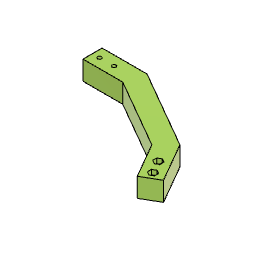
assembly (Autodesk Fusion 360 archive; units mm, degrees)
design "circular_frame"
Autodesk Fusion 360 part; units mm, degrees
(part 1 of 2)
sketch "Sketch1" plane through (0, 0, 0) normal (0, 0, 1) x (1, 0, 0)
  line L0 (151.5544, -62.5) -> (128.1089, -21.8911)
  line L1 (128.1089, -21.8911) -> (46.8911, 25)
  line L2 (46.8911, 25) -> (0, 25)
  line L3 (0, 0) -> (0, 25)
  arc A0 (129.9038, -75) -> (0, 0) centre (0, -150) ccw
  line L4 (151.5544, -62.5) -> (129.9038, -75)
  line L5 (113.4679, -36.5321) -> (41.5321, 5)
  line L6 (41.5321, 5) -> (0, 5)
  line L7 (134.2339, -72.5) -> (113.4679, -36.5321)
  line L8 (77.5, -15.7661) -> (87.5, 1.5544)
  point P0 (0, -150)
  point P1 (0, -150)
  dimension "d1" = 300
  dimension "d4" = 150
  dimension "d5" = 150
  dimension "d14" = 25
  dimension "d15" = 25
  dimension "d16" = 60
  dimension "d17" = 175
  dimension "d30" = 20
  dimension "d31" = 20
  dimension "d32" = 20
  constraint coincident L3.start A0
  constraint vertical L3.start A0.centre
  constraint coincident P0 A0.centre
  constraint horizontal L2
  constraint coincident L3.start A0.end
  constraint coincident L3 A0.end
  constraint collinear L3.start P1 L2.end
  constraint collinear P0 L0.start A0.start
  constraint coincident L3 L6.end
  constraint perpendicular L3 L6
  constraint parallel L1 L5
  constraint midpoint L5 L8.start
  constraint midpoint L1 L8.end
  measures "d1" diameter of A0
  measures "d4" angle of L1 L2
  measures "d5" angle of L0 L1
  measures "d14" distance of L3.start L2.end
  measures "d15" distance of L0.start A0.start
  measures "d16" angle of L3 L4
  measures "d17" distance of P0 L1
  measures "d30" distance of L0 L7
  measures "d31" distance of L2.end L6.end
  measures "d32" distance of L1 L5
extrude "Extrude1" add sketch "Sketch1" along normal blind 20 contours L1 L2 L3 L5 L6 L8
mirror "Mirror2" about plane through (77.5, -15.7661, 0) normal (0.866025, -0.5, 0) of bodies 1 merged
sketch "Sketch4" plane through (0, 0, 20) normal (0, 0, 1) x (-1, 0, 0)
  line L0 (-128.1089, 21.8911) -> (-46.8911, -25)
  line L1 (-46.8911, -25) -> (0, -25)
  line L2 (-41.5321, -5) -> (-41.5321, -25) construction
  line L3 (-41.5321, -15) -> (0, -15) construction
  circle A0 centre (-7.5, -15) radius 2
  circle A1 centre (-22.5, -15) radius 2
  line L4 (-3.8, -17.1362) -> (-3.8, -12.8638)
  line L5 (-3.8, -12.8638) -> (-7.5, -10.7276)
  line L6 (-7.5, -10.7276) -> (-11.2, -12.8638)
  line L7 (-11.2, -12.8638) -> (-11.2, -17.1362)
  line L8 (-11.2, -17.1362) -> (-7.5, -19.2724)
  line L9 (-7.5, -19.2724) -> (-3.8, -17.1362)
  line L10 (-18.8, -17.1362) -> (-18.8, -12.8638)
  line L11 (-18.8, -12.8638) -> (-22.5, -10.7276)
  line L12 (-22.5, -10.7276) -> (-26.2, -12.8638)
  line L13 (-26.2, -12.8638) -> (-26.2, -17.1362)
  line L14 (-26.2, -17.1362) -> (-22.5, -19.2724)
  line L15 (-22.5, -19.2724) -> (-18.8, -17.1362)
  line L16 (0, -5) -> (-41.5321, -5)
  line L17 (-41.5321, -5) -> (-113.4679, 36.5321)
  line L18 (0, -25) -> (0, -5)
  line L19 (-113.4679, 36.5321) -> (-134.2339, 72.5)
  line L20 (-134.2339, 72.5) -> (-151.5544, 62.5)
  line L21 (-151.5544, 62.5) -> (-128.1089, 21.8911)
  line L22 (-77.5, 15.7661) -> (-87.5, -1.5544) construction
  line L23 (-142.8442, 58.8686) -> (-142.8442, 63.141)
  line L24 (-139.1442, 56.7324) -> (-142.8442, 58.8686)
  line L25 (-135.4442, 58.8686) -> (-139.1442, 56.7324)
  line L26 (-135.4442, 63.141) -> (-135.4442, 58.8686)
  line L27 (-139.1442, 65.2772) -> (-135.4442, 63.141)
  line L28 (-142.8442, 63.141) -> (-139.1442, 65.2772)
  line L29 (-131.6442, 52.2868) -> (-127.9442, 50.1506)
  line L30 (-135.3442, 50.1506) -> (-131.6442, 52.2868)
  line L31 (-135.3442, 45.8782) -> (-135.3442, 50.1506)
  line L32 (-131.6442, 43.742) -> (-135.3442, 45.8782)
  line L33 (-127.9442, 45.8782) -> (-131.6442, 43.742)
  line L34 (-127.9442, 50.1506) -> (-127.9442, 45.8782)
  circle A2 centre (-139.1442, 61.0048) radius 2
  circle A3 centre (-131.6442, 48.0144) radius 2
  point P0 (-7.5, -15)
  point P1 (-22.5, -15)
  dimension "d18" = 4
  dimension "d19" = 7.5
  dimension "d20" = 15
  dimension "d21" = 7.4
  constraint coincident L1 L2.end
  constraint perpendicular L1 L2
  constraint midpoint L2 L3.start
  constraint coincident L3 P0
  constraint coincident L3 P1
  constraint equal A0 A1
  constraint coincident P0 A0.centre
  constraint coincident P1 A1.centre
  constraint vertical L4
  constraint vertical L10
  constraint horizontal L8.end L14.end
  constraint horizontal L3
  constraint coincident L2.start L16
  constraint coincident L3.end L18
  constraint coincident L2.start L16.end
  constraint midpoint L17 L22.start
  constraint midpoint L0 L22.end
  constraint symmetric L4.start L22 L23.end
  constraint symmetric L4.end L22 L27.start
  constraint symmetric L5.end L22 L26.start
  constraint symmetric L6.end L22 L25.start
  constraint symmetric L7.end L22 L24.start
  constraint symmetric L8.end L22 L23.start
  constraint symmetric L10.start L22 L30.start
  constraint symmetric L10.end L22 L29.start
  constraint symmetric L11.end L22 L29.end
  constraint symmetric L12.end L22 L33.start
  constraint symmetric L13.end L22 L32.start
  constraint symmetric L14.end L22 L31.start
  constraint symmetric A0 L22 A2
  constraint symmetric A1 L22 A3
  measures "d18" diameter of A0
  measures "d19" distance of L3.end P0
  measures "d20" distance of P0 P1
  measures "d21" distance of L4 L7
extrude "Extrude4" cut sketch "Sketch4" against normal through all contours A0 | A1 | A2 | A3
extrude "Extrude5" cut sketch "Sketch4" along normal blind 5 from surface at -20 contours L4 L5 L6 L7 L8 L9 | L10 L11 L12 L13 L14 L15
extrude "Extrude6" cut sketch "Sketch4" against normal blind 5 contours L23 L24 L25 L26 L27 L28 | L29 L30 L31 L32 L33 L34
equation "d21 = 7 mm + 2 * gap"
equation "gap = 0.2 mm"

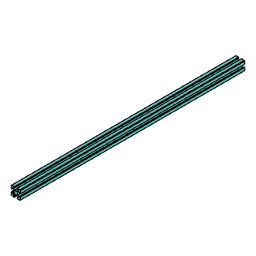
design "profile"
Autodesk Fusion 360 part; units mm, degrees
sketch "Sketch1" plane through (0, 0, 0) normal (0, 1, 0) x (1, 0, 0)
  line L0 (3.5, 0) -> (3.5, -2.7929)
  line L1 (3.5, -2.7929) -> (5.7071, -5)
  line L2 (5.7071, -5) -> (8, -5)
  line L3 (10, -3) -> (10, -10)
  line L4 (0, 0) -> (10, -10)
  line L5 (3.5, 0) -> (0, 0)
  line L6 (8, -5) -> (8, -3)
  line L7 (8, -3) -> (10, -3)
  dimension "d4" = 45
  dimension "d5" = 0.5
  dimension "d7" = 7
  dimension "d8" = 2
  dimension "d9" = 2
  dimension "d10" = 3.5
  dimension "d11" = 10
  constraint vertical L0
  constraint perpendicular L0 L2
  constraint perpendicular L2 L3
  constraint coincident L4.start L5.end
  constraint perpendicular L0 L5
  constraint parallel L1 L4
  constraint perpendicular L2 L6
  constraint horizontal L7
  measures "d4" angle of L4 L5
  measures "d5" distance of L1 L4
  measures "d7" distance of L3.start L3.end
  measures "d8" distance of L2.end L6.end
  measures "d9" distance of L3.start L6.end
  measures "d10" distance of L0.start L4.start
  measures "d11" distance of L4.start L3
extrude "Extrude1" add sketch "Sketch1" along normal blind 490
mirror "Mirror1" about plane through (0, 0, 0) normal (-0.707107, 0, 0.707107) of bodies 1 merged
mirror "Mirror2" about plane through (0, 0, 3.5) normal (-1, 0, 0) of bodies 1 merged
mirror "Mirror3" about plane through (3.5, 0, 0) normal (0, 0, -1) of bodies 1 merged
fillet "Fillet1" radius 1 4 edges at (-10, 245, 10) (10, 245, 10) (-10, 245, -10) (10, 245, -10)
sketch "Sketch2" plane through (0, 0, 0) normal (0, -1, 0) x (1, 0, 0)
  arc A0 (9, -10) -> (10, -9) centre (9, -9) ccw
  line L0 (10, -9) -> (10, -3)
  line L1 (10, -3) -> (8, -3)
  line L2 (8, -3) -> (8, -5)
  line L3 (8, -5) -> (5.7071, -5)
  line L4 (5.7071, -5) -> (3.5, -2.7929)
  line L5 (3.5, -2.7929) -> (3.5, 2.7929)
  line L6 (3.5, 2.7929) -> (5.7071, 5)
  line L7 (5.7071, 5) -> (8, 5)
  line L8 (8, 5) -> (8, 3)
  line L9 (8, 3) -> (10, 3)
  line L10 (10, 3) -> (10, 9)
  arc A1 (10, 9) -> (9, 10) centre (9, 9) ccw
  line L11 (9, 10) -> (3, 10)
  line L12 (3, 10) -> (3, 8)
  line L13 (3, 8) -> (5, 8)
  line L14 (5, 8) -> (5, 5.7071)
  line L15 (5, 5.7071) -> (2.7929, 3.5)
  line L16 (2.7929, 3.5) -> (-2.7929, 3.5)
  line L17 (-2.7929, 3.5) -> (-5, 5.7071)
  line L18 (-5, 5.7071) -> (-5, 8)
  line L19 (-5, 8) -> (-3, 8)
  line L20 (-3, 8) -> (-3, 10)
  line L21 (-3, 10) -> (-9, 10)
  arc A2 (-9, 10) -> (-10, 9) centre (-9, 9) ccw
  line L22 (-10, 9) -> (-10, 3)
  line L23 (-10, 3) -> (-8, 3)
  line L24 (-8, 3) -> (-8, 5)
  line L25 (-8, 5) -> (-5.7071, 5)
  line L26 (-5.7071, 5) -> (-3.5, 2.7929)
  line L27 (-3.5, 2.7929) -> (-3.5, -2.7929)
  line L28 (-3.5, -2.7929) -> (-5.7071, -5)
  line L29 (-5.7071, -5) -> (-8, -5)
  line L30 (-8, -5) -> (-8, -3)
  line L31 (-8, -3) -> (-10, -3)
  line L32 (-10, -3) -> (-10, -9)
  arc A3 (-10, -9) -> (-9, -10) centre (-9, -9) ccw
  line L33 (-9, -10) -> (-3, -10)
  line L34 (-3, -10) -> (-3, -8)
  line L35 (-3, -8) -> (-5, -8)
  line L36 (-5, -8) -> (-5, -5.7071)
  line L37 (-5, -5.7071) -> (-2.7929, -3.5)
  line L38 (-2.7929, -3.5) -> (2.7929, -3.5)
  line L39 (2.7929, -3.5) -> (5, -5.7071)
  line L40 (5, -5.7071) -> (5, -8)
  line L41 (5, -8) -> (3, -8)
  line L42 (3, -8) -> (3, -10)
  line L43 (3, -10) -> (9, -10)
  line L44 (2.9, 7.9) -> (4.9, 7.9)
  line L45 (4.9, 7.9) -> (4.9, 5.7485)
  line L46 (4.9, 5.7485) -> (2.7515, 3.6)
  line L47 (2.7515, 3.6) -> (-2.7515, 3.6)
  line L48 (-2.7515, 3.6) -> (-4.9, 5.7485)
  line L49 (-4.9, 5.7485) -> (-4.9, 7.9)
  line L50 (-4.9, 7.9) -> (-2.9, 7.9)
  line L51 (-2.9, 7.9) -> (-2.9, 10.1)
  line L52 (-2.9, 10.1) -> (-9, 10.1)
  arc A4 (-9, 10.1) -> (-10.1, 9) centre (-9, 9) ccw
  line L53 (-10.1, 9) -> (-10.1, 2.9)
  line L54 (-10.1, 2.9) -> (-7.9, 2.9)
  line L55 (-7.9, 2.9) -> (-7.9, 4.9)
  line L56 (-7.9, 4.9) -> (-5.7485, 4.9)
  line L57 (-5.7485, 4.9) -> (-3.6, 2.7515)
  line L58 (-3.6, 2.7515) -> (-3.6, -2.7515)
  line L59 (-3.6, -2.7515) -> (-5.7485, -4.9)
  line L60 (-5.7485, -4.9) -> (-7.9, -4.9)
  line L61 (-7.9, -4.9) -> (-7.9, -2.9)
  line L62 (-7.9, -2.9) -> (-10.1, -2.9)
  line L63 (-10.1, -2.9) -> (-10.1, -9)
  arc A5 (-10.1, -9) -> (-9, -10.1) centre (-9, -9) ccw
  line L64 (-9, -10.1) -> (-2.9, -10.1)
  line L65 (-2.9, -10.1) -> (-2.9, -7.9)
  line L66 (-2.9, -7.9) -> (-4.9, -7.9)
  line L67 (-4.9, -7.9) -> (-4.9, -5.7485)
  line L68 (-4.9, -5.7485) -> (-2.7515, -3.6)
  line L69 (-2.7515, -3.6) -> (2.7515, -3.6)
  line L70 (2.7515, -3.6) -> (4.9, -5.7485)
  line L71 (4.9, -5.7485) -> (4.9, -7.9)
  line L72 (4.9, -7.9) -> (2.9, -7.9)
  line L73 (2.9, -7.9) -> (2.9, -10.1)
  line L74 (2.9, -10.1) -> (9, -10.1)
  arc A6 (9, -10.1) -> (10.1, -9) centre (9, -9) ccw
  line L75 (10.1, -9) -> (10.1, -2.9)
  line L76 (10.1, -2.9) -> (7.9, -2.9)
  line L77 (7.9, -2.9) -> (7.9, -4.9)
  line L78 (7.9, -4.9) -> (5.7485, -4.9)
  line L79 (5.7485, -4.9) -> (3.6, -2.7515)
  line L80 (3.6, -2.7515) -> (3.6, 2.7515)
  line L81 (3.6, 2.7515) -> (5.7485, 4.9)
  line L82 (5.7485, 4.9) -> (7.9, 4.9)
  line L83 (7.9, 4.9) -> (7.9, 2.9)
  line L84 (7.9, 2.9) -> (10.1, 2.9)
  line L85 (10.1, 2.9) -> (10.1, 9)
  arc A7 (10.1, 9) -> (9, 10.1) centre (9, 9) ccw
  line L86 (9, 10.1) -> (2.9, 10.1)
  line L87 (2.9, 10.1) -> (2.9, 7.9)
  dimension "d22" = 0.1
sketch "Sketch3" plane through (0, 0, 0) normal (0, 1, 0) x (1, 0, 0)
  line L0 (10.1, 9) -> (10.1, 2.9)
  arc A0 (10.1, 9) -> (9, 10.1) centre (9, 9) ccw
  line L1 (2.9, 10.1) -> (9, 10.1)
  line L2 (2.9, 7.9) -> (2.9, 10.1)
  line L3 (4.9, 7.9) -> (2.9, 7.9)
  line L4 (4.9, 5.7485) -> (4.9, 7.9)
  line L5 (2.7515, 3.6) -> (4.9, 5.7485)
  line L6 (5.7485, 4.9) -> (3.6, 2.7515)
  line L7 (7.9, 4.9) -> (5.7485, 4.9)
  line L8 (7.9, 2.9) -> (7.9, 4.9)
  line L9 (10.1, 2.9) -> (7.9, 2.9)
  line L10 (3.6, 2.7515) -> (3.6, -2.7515)
  line L11 (3.6, -2.7515) -> (5.7485, -4.9)
  line L12 (5.7485, -4.9) -> (7.9, -4.9)
  line L13 (7.9, -4.9) -> (7.9, -2.9)
  line L14 (7.9, -2.9) -> (10.1, -2.9)
  line L15 (10.1, -2.9) -> (10.1, -9)
  arc A1 (9, -10.1) -> (10.1, -9) centre (9, -9) ccw
  line L16 (9, -10.1) -> (2.9, -10.1)
  line L17 (2.9, -10.1) -> (2.9, -7.9)
  line L18 (2.9, -7.9) -> (4.9, -7.9)
  line L19 (4.9, -7.9) -> (4.9, -5.7485)
  line L20 (4.9, -5.7485) -> (2.7515, -3.6)
  line L21 (2.7515, -3.6) -> (-2.7515, -3.6)
  line L22 (-2.7515, -3.6) -> (-4.9, -5.7485)
  line L23 (-4.9, -5.7485) -> (-4.9, -7.9)
  line L24 (-4.9, -7.9) -> (-2.9, -7.9)
  line L25 (-2.9, -7.9) -> (-2.9, -10.1)
  line L26 (-2.9, -10.1) -> (-9, -10.1)
  arc A2 (-10.1, -9) -> (-9, -10.1) centre (-9, -9) ccw
  line L27 (-10.1, -9) -> (-10.1, -2.9)
  line L28 (-10.1, -2.9) -> (-7.9, -2.9)
  line L29 (-7.9, -2.9) -> (-7.9, -4.9)
  line L30 (-7.9, -4.9) -> (-5.7485, -4.9)
  line L31 (-5.7485, -4.9) -> (-3.6, -2.7515)
  line L32 (-3.6, -2.7515) -> (-3.6, 2.7515)
  line L33 (-3.6, 2.7515) -> (-5.7485, 4.9)
  line L34 (-7.9, 2.9) -> (-10.1, 2.9)
  line L35 (-7.9, 4.9) -> (-7.9, 2.9)
  line L36 (-5.7485, 4.9) -> (-7.9, 4.9)
  line L37 (-10.1, 2.9) -> (-10.1, 9)
  line L38 (-4.9, 5.7485) -> (-2.7515, 3.6)
  line L39 (-2.7515, 3.6) -> (2.7515, 3.6)
  line L40 (-4.9, 7.9) -> (-4.9, 5.7485)
  line L41 (-2.9, 7.9) -> (-4.9, 7.9)
  line L42 (-2.9, 10.1) -> (-2.9, 7.9)
  line L43 (-9, 10.1) -> (-2.9, 10.1)
  arc A3 (-9, 10.1) -> (-10.1, 9) centre (-9, 9) ccw

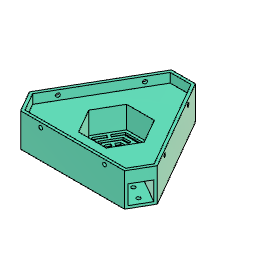
design "lower_connector"
Autodesk Fusion 360 part; units mm, degrees
sketch "Sketch1" plane through (0, 0, 0) normal (0, 0, 1) x (1, 0, 0)
  line L0 (-26, 0) -> (-82.282, -97.4833)
  line L1 (-69.282, -120) -> (43.282, -120)
  line L2 (56.282, -97.4833) -> (0, 0)
  line L3 (49.782, -108.7417) -> (-54.141, -48.7417) construction
  line L4 (0, 0) -> (-26, 0)
  line L5 (-82.282, -97.4833) -> (-69.282, -120)
  line L6 (43.282, -120) -> (56.282, -97.4833)
  line L7 (-13, 0) -> (-13, -120) construction
  line L8 (-75.782, -108.7417) -> (28.141, -48.7417) construction
  line L9 (-24.2679, -3) -> (-78.8179, -97.4833)
  line L10 (-78.8179, -97.4833) -> (-67.55, -117)
  line L11 (-67.55, -117) -> (41.55, -117)
  line L12 (41.55, -117) -> (52.8179, -97.4833)
  line L13 (52.8179, -97.4833) -> (-1.7321, -3)
  line L14 (-1.7321, -3) -> (-24.2679, -3)
  line L15 (2, -98.4752) -> (-28, -98.4752)
  line L16 (-28, -98.4752) -> (-43, -72.4944)
  line L17 (-43, -72.4944) -> (-28, -46.5137)
  line L18 (-28, -46.5137) -> (2, -46.5137)
  line L19 (2, -46.5137) -> (17, -72.4944)
  line L20 (17, -72.4944) -> (2, -98.4752)
  point P0 (-13, -72.4944)
  dimension "d18" = 120
  dimension "d25" = -3
  dimension "d36" = 26
  dimension "d42" = 30
  constraint coincident L2.end L4.start
  constraint horizontal L1
  constraint midpoint L0 L3.end
  constraint coincident L3 P0
  constraint symmetric L1.end L2.start L3
  constraint coincident L3.start L6
  constraint horizontal L4
  constraint midpoint L4 L7.start
  constraint midpoint L1 L7.end
  constraint midpoint L5 L8.start
  constraint midpoint L2 L8.end
  constraint coincident P0 L8
  constraint coincident P0 L7
  constraint perpendicular L4 L7
  constraint perpendicular L5 L8
  constraint symmetric L0 L1 L8
  constraint symmetric L0 L2 L7
  constraint equal L1 L2
  constraint horizontal L15
  constraint perpendicular L8 L16
  constraint parallel L15 L18
  constraint perpendicular L3 L20
  constraint perpendicular L8 L19
  constraint perpendicular L3 L17
  constraint symmetric L7 L16 L20
  constraint symmetric L7 L17 L19
  constraint symmetric L3 L16 L18
  constraint symmetric L3 L15 L19
  constraint equal L15 L16
  measures "d18" distance of L2.end L1
  measures "d36" distance of L1.end L2.start
  measures "d42" distance of L15.start L15.end
extrude "Extrude7" add sketch "Sketch1" along normal blind 2 contours L15 L16 L17 L18 L19 L20
extrude "Extrude4" add sketch "Sketch1" along normal blind 26 contours L0 L1 L2 L4 L5 L6 | L9 L10 L11 L12 L13 L14
sketch "Sketch2" plane through (84.423, -48.7417, 0) normal (0.866025, -0.5, 0) x (0.5, 0.866025, 0)
  line L0 (-82.282, 0) -> (-56.282, 0)
  line L1 (-56.282, 0) -> (-56.282, 26)
  line L2 (-56.282, 26) -> (-82.282, 26)
  line L3 (-82.282, 26) -> (-82.282, 0)
  line L4 (-82.282, 0) -> (-56.282, 26) construction
  line L5 (-56.282, 0) -> (-82.282, 26) construction
  line L6 (-79.482, 2.8) -> (-59.082, 2.8)
  line L7 (-59.082, 2.8) -> (-59.082, 23.2)
  line L8 (-59.082, 23.2) -> (-79.482, 23.2)
  line L9 (-79.482, 23.2) -> (-79.482, 2.8)
  dimension "d79" = 20.4
  constraint coincident L0.start L3.end
  constraint coincident L1.end L2.start
  constraint coincident L0.end L1.start
  constraint coincident L2.end L3.start
  constraint horizontal L6
  constraint vertical L7
  constraint horizontal L8
  constraint vertical L9
  constraint coincident L4 L7.end
  constraint coincident L4 L6.start
  constraint coincident L5 L8.end
  measures "d79" distance of L7.end L8.end
extrude "Extrude5" cut sketch "Sketch2" against normal blind 30 contours L6 L7 L8 L9
sketch "Sketch8" plane through (0, 0, 0) normal (0, 1, 0) x (-1, 0, 0)
  line L0 (0, 0) -> (26, 0)
  line L1 (26, 0) -> (26, 26)
  line L2 (26, 26) -> (0, 26)
  line L3 (0, 26) -> (0, 0)
  line L4 (0, 0) -> (26, 26) construction
  line L5 (0, 26) -> (26, 0) construction
  line L6 (2.8, 2.8) -> (23.2, 2.8)
  line L7 (23.2, 2.8) -> (23.2, 23.2)
  line L8 (23.2, 23.2) -> (2.8, 23.2)
  line L9 (2.8, 23.2) -> (2.8, 2.8)
  dimension "d62" = 20.4
  constraint coincident L0.start L3.end
  constraint coincident L1.end L2.start
  constraint coincident L2.end L3.start
  constraint coincident L0.end L1.start
  constraint horizontal L6
  constraint vertical L7
  constraint horizontal L8
  constraint vertical L9
  constraint coincident L4 L7.end
  constraint coincident L4 L6.start
  constraint coincident L5 L8.end
  measures "d62" distance of L7.end L8.end
extrude "Extrude9" cut sketch "Sketch8" against normal blind 30 contours L6 L7 L8 L9
sketch "Sketch9" plane through (-103.923, -60, 0) normal (-0.866025, -0.5, 0) x (0.5, -0.866025, 0)
  line L0 (43.282, 0) -> (69.282, 0)
  line L1 (69.282, 0) -> (69.282, 26)
  line L2 (69.282, 26) -> (43.282, 26)
  line L3 (43.282, 26) -> (43.282, 0)
  line L4 (43.282, 0) -> (69.282, 26) construction
  line L5 (43.282, 26) -> (69.282, 0) construction
  line L6 (46.082, 2.8) -> (66.482, 2.8)
  line L7 (66.482, 2.8) -> (66.482, 23.2)
  line L8 (66.482, 23.2) -> (46.082, 23.2)
  line L9 (46.082, 23.2) -> (46.082, 2.8)
  dimension "d65" = 20.4
  constraint coincident L0.start L3.end
  constraint coincident L1.end L2.start
  constraint coincident L2.end L3.start
  constraint coincident L0.end L1.start
  constraint horizontal L6
  constraint vertical L7
  constraint horizontal L8
  constraint vertical L9
  constraint coincident L4 L7.end
  constraint coincident L4 L6.start
  constraint coincident L5 L8.end
  measures "d65" distance of L7.end L8.end
extrude "Extrude10" cut sketch "Sketch9" against normal blind 30 contours L6 L7 L8 L9
sketch "Sketch7" plane through (0, 0, 2) normal (0, 0, 1) x (-1, 0, 0)
  line L0 (14.5, 80.4752, 24) -> (14.5, 83.4752, 24)
  line L1 (17.6077, 80.4752, 24) -> (14.5, 80.4752, 24)
  line L2 (24.3577, 80.7839, 24) -> (26.9558, 82.2839, 24)
  line L3 (18.7513, 72.4944, 24) -> (18.0635, 73.6858, 24)
  line L4 (25.6795, 72.4944, 24) -> (19.3397, 83.4752, 24)
  line L5 (22.2154, 72.4944, 24) -> (20.6615, 75.1858, 24)
  line L6 (19.1615, 77.7839, 24) -> (17.6077, 80.4752, 24)
  line L7 (24.3577, 80.7839, 24) -> (21.0718, 86.4752, 24)
  line L8 (20.6615, 75.1858, 24) -> (19.1615, 77.7839, 24)
  line L9 (19.3397, 83.4752, 24) -> (14.5, 83.4752, 24)
  line L10 (18.0635, 73.6858, 24) -> (20.6615, 75.1858, 24)
  line L11 (25.8577, 78.1858, 24) -> (28.4558, 79.6858, 24)
  line L12 (16.5635, 76.2839, 24) -> (15.8756, 77.4752, 24)
  line L13 (18.0635, 73.6858, 24) -> (16.5635, 76.2839, 24)
  line L14 (15.8756, 77.4752, 24) -> (10.1244, 77.4752, 24)
  line L15 (16.5635, 76.2839, 24) -> (19.1615, 77.7839, 24)
  line L16 (26.2679, 95.4752, 24) -> (14.5, 95.4752, 24)
  line L17 (24.5359, 92.4752, 24) -> (14.5, 92.4752, 24)
  line L18 (29.1436, 72.4944, 24) -> (25.8577, 78.1858, 24)
  line L19 (6.6603, 61.5137, 24) -> (19.3397, 61.5137, 24)
  line L20 (26.9558, 82.2839, 24) -> (22.8038, 89.4752, 24)
  line L21 (14.5, 58.5137, 24) -> (21.0718, 58.5137, 24)
  line L22 (14.5, 55.5137, 24) -> (22.8038, 55.5137, 24)
  line L23 (11.5, 64.5137, 24) -> (14.5, 64.5137, 24)
  line L24 (14.5, 92.4752, 24) -> (14.5, 95.4752, 24)
  line L25 (19.3397, 61.5137, 24) -> (21.7596, 65.705, 24)
  line L26 (17.6077, 64.5137, 24) -> (19.1615, 67.205, 24)
  line L27 (32.6077, 72.4944, 24) -> (28.4558, 79.6858, 24)
  line L28 (34.75, 58.205, 24) -> (-10.25, 84.1858, 24) construction
  line L29 (4.2404, 65.705, 24) -> (2.7404, 68.3031, 24)
  line L30 (3.1962, 55.5137, 24) -> (11.5, 55.5137, 24)
  line L31 (10.1244, 67.5137, 24) -> (11.5, 67.5137, 24)
  line L32 (5.3385, 69.8031, 24) -> (2.7404, 68.3031, 24)
  line L33 (3.7846, 72.4944, 24) -> (5.3385, 69.8031, 24)
  line L34 (7.2487, 72.4944, 24) -> (10.1244, 67.5137, 24)
  line L35 (-0.2679, 49.5137, 24) -> (26.2679, 49.5137, 24)
  line L36 (0.3205, 72.4944, 24) -> (2.7404, 68.3031, 24)
  line L37 (6.8385, 67.205, 24) -> (5.3385, 69.8031, 24)
  line L38 (-13.5359, 72.4944, 24) -> (-7.6519, 62.3031, 24)
  line L39 (-2, 46.5137, 24) -> (28, 46.5137, 24)
  line L40 (-2, 98.4752, 24) -> (-17, 72.4944, 24)
  line L41 (11.5, 98.4752, 24) -> (11.5, 46.5137, 24) construction
  line L42 (-6.6077, 72.4944, 24) -> (3.1962, 55.5137, 24)
  line L43 (-17, 72.4944, 24) -> (-2, 46.5137, 24)
  line L44 (11.5, 67.5137, 24) -> (11.5, 64.5137, 24)
  line L45 (8.3923, 64.5137, 24) -> (11.5, 64.5137, 24)
  line L46 (34.75, 86.7839, 24) -> (-10.25, 60.8031, 24) construction
  line L47 (11.5, 58.5137, 24) -> (11.5, 55.5137, 24)
  line L48 (4.2404, 65.705, 24) -> (6.6603, 61.5137, 24)
  line L49 (6.8385, 67.205, 24) -> (4.2404, 65.705, 24)
  line L50 (6.8385, 67.205, 24) -> (8.3923, 64.5137, 24)
  line L51 (-3.5538, 61.205, 24) -> (1.4641, 52.5137, 24)
  line L52 (-9.5, 59.5041, 24) -> (35.5, 85.4848, 24) construction
  line L53 (4.9282, 58.5137, 24) -> (11.5, 58.5137, 24)
  line L54 (-10.0718, 72.4944, 24) -> (-5.0538, 63.8031, 24)
  line L55 (36.25, 84.1858, 24) -> (-8.75, 58.205, 24) construction
  line L56 (23.2596, 68.3031, 24) -> (25.6795, 72.4944, 24)
  line L57 (15.8756, 67.5137, 24) -> (18.7513, 72.4944, 24)
  line L58 (26.2679, 49.5137, 24) -> (32.1519, 59.705, 24)
  line L59 (31.0538, 63.8031, 24) -> (36.0718, 72.4944, 24)
  line L60 (22.8038, 55.5137, 24) -> (32.6077, 72.4944, 24)
  line L61 (19.1615, 67.205, 24) -> (21.7596, 65.705, 24)
  line L62 (36.0718, 72.4944, 24) -> (24.5359, 92.4752, 24)
  line L63 (14.5, 64.5137, 24) -> (17.6077, 64.5137, 24)
  line L64 (43, 72.4944, 24) -> (28, 98.4752, 24)
  line L65 (39.5359, 72.4944, 24) -> (26.2679, 95.4752, 24)
  line L66 (29.5538, 61.205, 24) -> (32.1519, 59.705, 24)
  line L67 (19.1615, 67.205, 24) -> (20.6615, 69.8031, 24)
  line L68 (21.7596, 65.705, 24) -> (23.2596, 68.3031, 24)
  line L69 (28, 46.5137, 24) -> (43, 72.4944, 24)
  line L70 (14.5, 67.5137, 24) -> (15.8756, 67.5137, 24)
  line L71 (11.5, 67.5137, 24) -> (14.5, 67.5137, 24)
  line L72 (14.5, 64.5137, 24) -> (14.5, 67.5137, 24)
  line L73 (23.2596, 68.3031, 24) -> (20.6615, 69.8031, 24)
  line L74 (14.5, 55.5137, 24) -> (14.5, 58.5137, 24)
  line L75 (14.5, 46.5137, 24) -> (14.5, 98.4752, 24) construction
  line L76 (21.0718, 58.5137, 24) -> (29.1436, 72.4944, 24)
  line L77 (24.5359, 52.5137, 24) -> (29.5538, 61.205, 24)
  line L78 (20.6615, 69.8031, 24) -> (22.2154, 72.4944, 24)
  line L79 (5.3385, 75.1858, 24) -> (6.8385, 77.7839, 24)
  line L80 (13, 98.4752, 24) -> (13, 46.5137, 24) construction
  line L81 (33.6519, 62.3031, 24) -> (39.5359, 72.4944, 24)
  line L82 (33.6519, 62.3031, 24) -> (31.0538, 63.8031, 24)
  line L83 (1.4641, 52.5137, 24) -> (24.5359, 52.5137, 24)
  line L84 (-3.1436, 72.4944, 24) -> (4.9282, 58.5137, 24)
  line L85 (36.25, 60.8031, 24) -> (-8.75, 86.7839, 24) construction
  line L86 (35.5, 59.5041, 24) -> (-9.5, 85.4848, 24) construction
  line L87 (1.4641, 92.4752, 24) -> (-10.0718, 72.4944, 24)
  line L88 (-0.2679, 95.4752, 24) -> (-13.5359, 72.4944, 24)
  line L89 (-3.5538, 61.205, 24) -> (-6.1519, 59.705, 24)
  line L90 (22.8038, 89.4752, 24) -> (3.1962, 89.4752, 24)
  line L91 (11.5, 83.4752, 24) -> (6.6603, 83.4752, 24)
  line L92 (8.3923, 80.4752, 24) -> (6.8385, 77.7839, 24)
  line L93 (5.3385, 75.1858, 24) -> (3.7846, 72.4944, 24)
  line L94 (28, 98.4752, 24) -> (-2, 98.4752, 24)
  line L95 (3.1962, 89.4752, 24) -> (-0.9558, 82.2839, 24)
  line L96 (11.5, 92.4752, 24) -> (1.4641, 92.4752, 24)
  line L97 (-5.0538, 63.8031, 24) -> (-7.6519, 62.3031, 24)
  line L98 (11.5, 83.4752, 24) -> (11.5, 80.4752, 24)
  line L99 (21.0718, 86.4752, 24) -> (4.9282, 86.4752, 24)
  line L100 (-6.1519, 59.705, 24) -> (-0.2679, 49.5137, 24)
  line L101 (4.9282, 86.4752, 24) -> (1.6423, 80.7839, 24)
  line L102 (-2.4558, 79.6858, 24) -> (-6.6077, 72.4944, 24)
  line L103 (-2.4558, 79.6858, 24) -> (0.1423, 78.1858, 24)
  line L104 (11.5, 95.4752, 24) -> (-0.2679, 95.4752, 24)
  line L105 (2.7404, 76.6858, 24) -> (0.3205, 72.4944, 24)
  line L106 (4.2404, 79.2839, 24) -> (2.7404, 76.6858, 24)
  line L107 (7.9365, 73.6858, 24) -> (7.2487, 72.4944, 24)
  line L108 (11.5, 95.4752, 24) -> (11.5, 92.4752, 24)
  line L109 (10.1244, 77.4752, 24) -> (9.4365, 76.2839, 24)
  line L110 (1.6423, 80.7839, 24) -> (-0.9558, 82.2839, 24)
  line L111 (11.5, 80.4752, 24) -> (8.3923, 80.4752, 24)
  line L112 (9.4365, 76.2839, 24) -> (6.8385, 77.7839, 24)
  line L113 (7.9365, 73.6858, 24) -> (5.3385, 75.1858, 24)
  line L114 (7.9365, 73.6858, 24) -> (9.4365, 76.2839, 24)
  line L115 (0.1423, 78.1858, 24) -> (-3.1436, 72.4944, 24)
  line L116 (6.6603, 83.4752, 24) -> (4.2404, 79.2839, 24)
  dimension "d80" = 3
  dimension "d81" = 3
  dimension "d82" = 3
  dimension "d83" = 3
  dimension "d84" = 3
  dimension "d85" = 3
  dimension "d86" = 6
  dimension "d87" = 6
  dimension "d88" = 6
  dimension "d89" = 6
  dimension "d90" = 6
  dimension "d91" = 6
  dimension "d92" = 9
  dimension "d93" = 9
  dimension "d94" = 9
  dimension "d95" = 9
  dimension "d96" = 9
  dimension "d97" = 9
  dimension "d98" = 12
  dimension "d99" = 12
  dimension "d100" = 12
  dimension "d101" = 12
  dimension "d102" = 12
  dimension "d103" = 12
  dimension "d104" = 18
  dimension "d105" = 18
  dimension "d106" = 18
  dimension "d107" = 18
  dimension "d108" = 18
  dimension "d109" = 18
  dimension "d110" = 15
  dimension "d111" = 15
  dimension "d112" = 15
  dimension "d113" = 15
  dimension "d114" = 15
  dimension "d115" = 15
  dimension "d116" = 3
  dimension "d117" = 3
  dimension "d118" = 3
  dimension "d119" = 21
  dimension "d120" = 21
  dimension "d121" = 21
  dimension "d122" = 21
  dimension "d123" = 21
  dimension "d124" = 21
extrude "Extrude8" cut sketch "Sketch7" against normal blind 65 contours L0 L1 L4 L5 L6 L8 L9 L56 L73 L78 | L3 L12 L13 L14 L31 L34 L57 L70 L71 L107 L109 L114 | L19 L23 L25 L26 L45 L48 L49 L50 L61 L63 | L32 L33 L36 L79 L91 L92 L93 L98 L105 L106 L111 L116 | L2 L7 L20 L90 L95 L99 L101 L110 | L11 L18 L21 L22 L27 L60 L74 L76 | L16 L17 L24 L59 L62 L65 L81 L82 | L30 L42 L47 L53 L84 L102 L103 L115 | L35 L51 L58 L66 L77 L83 L89 L100 | L38 L54 L87 L88 L96 L97 L104 L108 in plane through (0, 0, 26) normal (0, 0, 1)
sketch "Sketch13" plane through (0, 0, 0) normal (0, 0, -1) x (1, 0, 0)
  line L0 (-6.6603, 83.4752) -> (-0.3205, 72.4944)
  line L1 (-0.3205, 72.4944) -> (-2.7404, 68.3031)
  line L2 (-2.7404, 68.3031) -> (-5.3385, 69.8031)
  line L3 (-5.3385, 69.8031) -> (-3.7846, 72.4944)
  line L4 (-3.7846, 72.4944) -> (-8.3923, 80.4752)
  line L5 (-8.3923, 80.4752) -> (-11.5, 80.4752)
  line L6 (-11.5, 80.4752) -> (-11.5, 83.4752)
  line L7 (-11.5, 83.4752) -> (-6.6603, 83.4752)
  line L8 (6.6077, 72.4944) -> (-3.1962, 55.5137)
  line L9 (-3.1962, 55.5137) -> (-11.5, 55.5137)
  line L10 (-11.5, 55.5137) -> (-11.5, 58.5137)
  line L11 (-11.5, 58.5137) -> (-4.9282, 58.5137)
  line L12 (-4.9282, 58.5137) -> (3.1436, 72.4944)
  line L13 (3.1436, 72.4944) -> (-0.1423, 78.1858)
  line L14 (-0.1423, 78.1858) -> (2.4558, 79.6858)
  line L15 (2.4558, 79.6858) -> (6.6077, 72.4944)
  line L16 (-26.2679, 95.4752) -> (-14.5, 95.4752)
  line L17 (-14.5, 95.4752) -> (-14.5, 92.4752)
  line L18 (-14.5, 92.4752) -> (-24.5359, 92.4752)
  line L19 (-24.5359, 92.4752) -> (-36.0718, 72.4944)
  line L20 (-36.0718, 72.4944) -> (-31.0538, 63.8031)
  line L21 (-31.0538, 63.8031) -> (-33.6519, 62.3031)
  line L22 (-33.6519, 62.3031) -> (-39.5359, 72.4944)
  line L23 (-39.5359, 72.4944) -> (-26.2679, 95.4752)
  line L24 (6.1519, 59.705) -> (0.2679, 49.5137)
  line L25 (0.2679, 49.5137) -> (-26.2679, 49.5137)
  line L26 (-26.2679, 49.5137) -> (-32.1519, 59.705)
  line L27 (-32.1519, 59.705) -> (-29.5538, 61.205)
  line L28 (-29.5538, 61.205) -> (-24.5359, 52.5137)
  line L29 (-24.5359, 52.5137) -> (-1.4641, 52.5137)
  line L30 (-1.4641, 52.5137) -> (3.5538, 61.205)
  line L31 (3.5538, 61.205) -> (6.1519, 59.705)
  line L32 (-4.2404, 65.705) -> (-6.6603, 61.5137)
  line L33 (-6.6603, 61.5137) -> (-19.3397, 61.5137)
  line L34 (-19.3397, 61.5137) -> (-21.7596, 65.705)
  line L35 (-21.7596, 65.705) -> (-19.1615, 67.205)
  line L36 (-19.1615, 67.205) -> (-17.6077, 64.5137)
  line L37 (-17.6077, 64.5137) -> (-8.3923, 64.5137)
  line L38 (-8.3923, 64.5137) -> (-6.8385, 67.205)
  line L39 (-6.8385, 67.205) -> (-4.2404, 65.705)
  line L40 (-25.6795, 72.4944) -> (-19.3397, 83.4752)
  line L41 (-19.3397, 83.4752) -> (-14.5, 83.4752)
  line L42 (-14.5, 83.4752) -> (-14.5, 80.4752)
  line L43 (-14.5, 80.4752) -> (-17.6077, 80.4752)
  line L44 (-17.6077, 80.4752) -> (-22.2154, 72.4944)
  line L45 (-22.2154, 72.4944) -> (-20.6615, 69.8031)
  line L46 (-20.6615, 69.8031) -> (-23.2596, 68.3031)
  line L47 (-23.2596, 68.3031) -> (-25.6795, 72.4944)
  line L48 (-26.9558, 82.2839) -> (-22.8038, 89.4752)
  line L49 (-22.8038, 89.4752) -> (-3.1962, 89.4752)
  line L50 (-3.1962, 89.4752) -> (0.9558, 82.2839)
  line L51 (0.9558, 82.2839) -> (-1.6423, 80.7839)
  line L52 (-1.6423, 80.7839) -> (-4.9282, 86.4752)
  line L53 (-4.9282, 86.4752) -> (-21.0718, 86.4752)
  line L54 (-21.0718, 86.4752) -> (-24.3577, 80.7839)
  line L55 (-24.3577, 80.7839) -> (-26.9558, 82.2839)
  line L56 (13.5359, 72.4944) -> (7.6519, 62.3031)
  line L57 (7.6519, 62.3031) -> (5.0538, 63.8031)
  line L58 (5.0538, 63.8031) -> (10.0718, 72.4944)
  line L59 (10.0718, 72.4944) -> (-1.4641, 92.4752)
  line L60 (-1.4641, 92.4752) -> (-11.5, 92.4752)
  line L61 (-11.5, 92.4752) -> (-11.5, 95.4752)
  line L62 (-11.5, 95.4752) -> (0.2679, 95.4752)
  line L63 (0.2679, 95.4752) -> (13.5359, 72.4944)
  line L64 (-22.8038, 55.5137) -> (-32.6077, 72.4944)
  line L65 (-32.6077, 72.4944) -> (-28.4558, 79.6858)
  line L66 (-28.4558, 79.6858) -> (-25.8577, 78.1858)
  line L67 (-25.8577, 78.1858) -> (-29.1436, 72.4944)
  line L68 (-29.1436, 72.4944) -> (-21.0718, 58.5137)
  line L69 (-21.0718, 58.5137) -> (-14.5, 58.5137)
  line L70 (-14.5, 58.5137) -> (-14.5, 55.5137)
  line L71 (-14.5, 55.5137) -> (-22.8038, 55.5137)
  line L72 (-10.1244, 67.5137) -> (-15.8756, 67.5137)
  line L73 (-15.8756, 67.5137) -> (-18.7513, 72.4944)
  line L74 (-18.7513, 72.4944) -> (-15.8756, 77.4752)
  line L75 (-15.8756, 77.4752) -> (-10.1244, 77.4752)
  line L76 (-10.1244, 77.4752) -> (-7.2487, 72.4944)
  line L77 (-7.2487, 72.4944) -> (-10.1244, 67.5137)
  line L78 (56.282, 97.4833) -> (43.282, 120)
  line L79 (43.282, 120) -> (-69.282, 120)
  line L80 (-69.282, 120) -> (-82.282, 97.4833)
  line L81 (-82.282, 97.4833) -> (-26, 0)
  line L82 (-26, 0) -> (0, 0)
  line L83 (0, 0) -> (56.282, 97.4833)
  line L84 (-13, 0) -> (-13, 72.4944) construction
  line L85 (-13, 72.4944) -> (49.782, 108.7417) construction
  line L86 (-13, 72.4944) -> (-75.782, 108.7417) construction
  circle A0 centre (-13, 7.5) radius 2
  circle A1 centre (-13, 22.5) radius 2
  circle A2 centre (43.2868, 104.9917) radius 2
  circle A3 centre (30.2965, 97.4917) radius 2
  circle A4 centre (-69.2868, 104.9917) radius 2
  circle A5 centre (-56.2965, 97.4917) radius 2
  dimension "d136" = 4
  dimension "d137" = 7.5
  dimension "d138" = 15
  dimension "d139" = 7.5
  dimension "d140" = 15
  dimension "d141" = 7.5
  dimension "d142" = 15
  constraint midpoint L82 L84.start
  constraint perpendicular L82 L84
  constraint midpoint L78 L85.end
  constraint midpoint L80 L86.end
  constraint perpendicular L80 L86
  constraint coincident L84 A0.centre
  constraint coincident L84 A1.centre
  constraint coincident L85 A2.centre
  constraint coincident L85 A3.centre
  constraint coincident L86 A4.centre
  constraint coincident L86 A5.centre
  constraint equal A0 A1
  constraint equal A1 A5
  constraint equal A4 A5
  constraint equal A3 A4
  constraint equal A2 A3
  measures "d136" diameter of A2
  measures "d137" distance of L78 A2.centre
  measures "d138" distance of A2.centre A3.centre
  measures "d139" distance of L82 A0.centre
  measures "d140" distance of A0.centre A1.centre
  measures "d141" distance of L80 A4.centre
  measures "d142" distance of A4.centre A5.centre
extrude "Extrude14" cut sketch "Sketch13" against normal blind 10 contours A0 | A1 | A2 | A3 | A4 | A5
extrude "Extrude16" add sketch "Sketch1" along normal blind 10 from surface at 26 contours L0 L1 L2 L4 L5 L6
sketch "Sketch17" plane through (-16.9019, 9.7583, 0) normal (0.866025, -0.5, 0) x (0.5, 0.866025, 0)
  line L0 (-123.832, 26) -> (-14.7321, 26)
  line L1 (-14.7321, 26) -> (-14.7321, 36)
  line L2 (-14.7321, 36) -> (-123.832, 36)
  line L3 (-123.832, 36) -> (-123.832, 26)
  line L4 (-123.832, 31) -> (-14.7321, 31) construction
  line L5 (-69.282, 26) -> (-69.282, 36) construction
  circle A0 centre (-103.832, 31) radius 2
  circle A1 centre (-34.7321, 31) radius 2
  dimension "d154" = 20
  dimension "d155" = 4
  constraint midpoint L3 L4.start
  constraint midpoint L1 L4.end
  constraint midpoint L0 L5.start
  constraint midpoint L2 L5.end
  constraint coincident L4 A0.centre
  constraint coincident L4 A1.centre
  constraint equal A0 A1
  constraint symmetric L5 A0 A1
  measures "d154" distance of L4.start A0.centre
  measures "d155" diameter of A0
sketch "Sketch19" plane through (-2.5981, -1.5, 0) normal (-0.866025, -0.5, 0) x (0.5, -0.866025, 0)
  line L0 (1.7321, 26) -> (110.832, 26)
  line L1 (110.832, 26) -> (110.832, 36)
  line L2 (110.832, 36) -> (1.7321, 36)
  line L3 (1.7321, 36) -> (1.7321, 26)
  line L4 (1.7321, 31) -> (110.832, 31) construction
  line L5 (56.282, 26) -> (56.282, 36) construction
  circle A0 centre (90.832, 31) radius 2
  circle A1 centre (21.7321, 31) radius 2
  dimension "d156" = 20
  dimension "d157" = 4
  constraint coincident A1.centre L4
  constraint coincident A0.centre L4
  constraint equal A0 A1
  constraint symmetric L5 A0 A1
  constraint coincident L3 L4.start
  constraint coincident L2 L5.end
  constraint coincident L0 L5.start
  constraint coincident L1 L4.end
  constraint midpoint L1 L4.end
  constraint midpoint L2 L5.end
  constraint midpoint L0 L5.start
  measures "d156" distance of A1.centre L4.start
  measures "d157" diameter of A1
sketch "Sketch20" plane through (0, -117, 0) normal (0, 1, 0) x (-1, 0, 0)
  line L0 (-41.55, 26) -> (67.55, 26)
  line L1 (67.55, 26) -> (67.55, 36)
  line L2 (67.55, 36) -> (-41.55, 36)
  line L3 (-41.55, 36) -> (-41.55, 26)
  line L4 (-41.55, 31) -> (67.55, 31) construction
  line L5 (13, 26) -> (13, 36) construction
  circle A0 centre (47.55, 31) radius 2
  circle A1 centre (-21.55, 31) radius 2
  dimension "d158" = 20
  dimension "d159" = 4
  constraint coincident A1.centre L4
  constraint coincident A0.centre L4
  constraint equal A0 A1
  constraint symmetric L5 A0 A1
  constraint midpoint L3 L4.start
  constraint midpoint L0 L5.start
  constraint midpoint L2 L5.end
  constraint midpoint L1 L4.end
  measures "d158" distance of A1.centre L4.start
  measures "d159" diameter of A1
extrude "Extrude17" cut sketch "Sketch20" against normal blind 5 contours A0 | A1
extrude "Extrude18" cut sketch "Sketch19" against normal blind 5 contours A0 | A1
extrude "Extrude19" cut sketch "Sketch17" against normal blind 5 contours A0 | A1
equation "gap = 0.2 mm"
equation "d62 = 20 mm + 2 * gap"
equation "d65 = 20 mm + 2 * gap"
equation "d79 = 20 mm + 2 * gap"

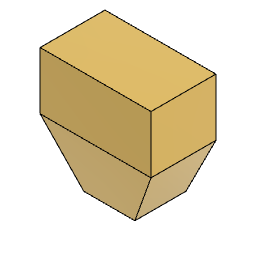
design "upper_single_connector"
Autodesk Fusion 360 part; units mm, degrees
sketch "Sketch1" plane through (0, 0, 0) normal (0, 1, 0) x (1, 0, 0)
  line L0 (7.9, 2.9) -> (7.9, 4.9)
  line L1 (-2.7515, -3.6) -> (-4.9, -5.7485)
  line L2 (2.9, -7.9) -> (4.9, -7.9)
  line L3 (-2.9, -7.9) -> (-2.9, -10.1)
  arc A0 (-10.1, -9) -> (-9, -10.1) centre (-9, -9) ccw
  line L4 (5.7485, 4.9) -> (3.6, 2.7515)
  line L5 (-7.9, 2.9) -> (-10.1, 2.9)
  line L6 (-4.9, -7.9) -> (-2.9, -7.9)
  line L7 (4.9, 5.7485) -> (4.9, 7.9)
  line L8 (10.1, 2.9) -> (7.9, 2.9)
  line L9 (9, -10.1) -> (2.9, -10.1)
  arc A1 (9, -10.1) -> (10.1, -9) centre (9, -9) ccw
  line L10 (4.9, -5.7485) -> (2.7515, -3.6)
  line L11 (5.7485, -4.9) -> (7.9, -4.9)
  line L12 (-10.1, 2.9) -> (-10.1, 9)
  line L13 (7.9, -2.9) -> (10.1, -2.9)
  line L14 (-3.6, 2.7515) -> (-5.7485, 4.9)
  line L15 (10.1, -2.9) -> (10.1, -9)
  line L16 (-2.9, 10.1) -> (-2.9, 7.9)
  line L17 (7.9, -4.9) -> (7.9, -2.9)
  line L18 (-3.6, -2.7515) -> (-3.6, 2.7515)
  line L19 (3.6, 2.7515) -> (3.6, -2.7515)
  line L20 (2.7515, -3.6) -> (-2.7515, -3.6)
  line L21 (-10.1, -9) -> (-10.1, -2.9)
  line L22 (10.1, 9) -> (10.1, 2.9)
  line L23 (2.9, 7.9) -> (2.9, 10.1)
  line L24 (7.9, 4.9) -> (5.7485, 4.9)
  line L25 (-2.9, -10.1) -> (-9, -10.1)
  line L26 (-2.7515, 3.6) -> (2.7515, 3.6)
  arc A2 (-9, 10.1) -> (-10.1, 9) centre (-9, 9) ccw
  line L27 (4.9, 7.9) -> (2.9, 7.9)
  line L28 (-7.9, -4.9) -> (-5.7485, -4.9)
  line L29 (2.9, 10.1) -> (9, 10.1)
  arc A3 (10.1, 9) -> (9, 10.1) centre (9, 9) ccw
  line L30 (-4.9, -5.7485) -> (-4.9, -7.9)
  line L31 (-7.9, -2.9) -> (-7.9, -4.9)
  line L32 (-4.9, 7.9) -> (-4.9, 5.7485)
  line L33 (2.7515, 3.6) -> (4.9, 5.7485)
  line L34 (-4.9, 5.7485) -> (-2.7515, 3.6)
  line L35 (-10.1, -2.9) -> (-7.9, -2.9)
  line L36 (3.6, -2.7515) -> (5.7485, -4.9)
  line L37 (4.9, -7.9) -> (4.9, -5.7485)
  line L38 (2.9, -10.1) -> (2.9, -7.9)
  line L39 (-5.7485, -4.9) -> (-3.6, -2.7515)
  line L40 (-7.9, 4.9) -> (-7.9, 2.9)
  line L41 (-2.9, 7.9) -> (-4.9, 7.9)
  line L42 (-9, 10.1) -> (-2.9, 10.1)
  line L43 (-5.7485, 4.9) -> (-7.9, 4.9)
  line L44 (-15.1, -14.6) -> (13.1, -14.6)
  line L45 (13.1, -14.6) -> (13.1, 14.6)
  line L46 (13.1, 14.6) -> (-15.1, 14.6)
  line L47 (-15.1, 14.6) -> (-15.1, -14.6)
  dimension "d1" = 3
  dimension "d2" = 5
  dimension "d3" = 4.5
  dimension "d4" = 4.5
  constraint horizontal L44
  constraint vertical L45
  constraint horizontal L46
  constraint vertical L47
  measures "d1" distance of L15 L45
  measures "d2" distance of L21 L47
  measures "d3" distance of L9 L44
  measures "d4" distance of L29 L46
extrude "Extrude1" add sketch "Sketch1" along normal blind 3 contours L0 L1 L2 L3 A0 L4 L5 L6 L7 L8 L9 A1 L10 L11 L12 L13 L14 L15 L16 L17 L18 L19 L20 L21 L22 L23 L24 L25 L26 A2 L27 L28 L29 A3 L30 L31 L32 L33 L34 L35 L36 L37 L38 L39 L40 L41 L42 L43 | L44 L45 L46 L47
extrude "Extrude2" add sketch "Sketch1" along normal blind 30 from surface at 3
mirror "Mirror1" about plane through (-15.1, 0, -14.6) normal (-1, 0, 0) of bodies 1 merged
ref_plane "WorkPlane1" through (-15.1, 16.5, -44.6) normal (0, 0, -1) x (-1, 0, 0)
sketch "Sketch2" plane through (0, 0, -44.6) normal (0, 0, -1) x (-1, 0, 0)
  line L0 (-13.1, 0) -> (43.3, 0)
  line L1 (43.3, 0) -> (43.3, 33)
  line L2 (43.3, 33) -> (-13.1, 33)
  line L3 (-13.1, 33) -> (-13.1, 0)
  line L4 (28.1, 33) -> (2.1, 33)
  line L5 (2.1, 33) -> (2.1, 7)
  line L6 (2.1, 7) -> (28.1, 7)
  line L7 (28.1, 7) -> (28.1, 33)
  line L8 (15.1, 33) -> (15.1, 0) construction
  line L9 (25.3, 30.2) -> (4.9, 30.2)
  line L10 (4.9, 30.2) -> (4.9, 9.8)
  line L11 (4.9, 9.8) -> (25.3, 9.8)
  line L12 (25.3, 9.8) -> (25.3, 30.2)
  dimension "d15" = 20.4
  dimension "d17" = 2.8
  dimension "d18" = 2.8
  dimension "d29" = 2.8
  constraint horizontal L4
  constraint vertical L5
  constraint horizontal L6
  constraint vertical L7
  constraint coincident L2 L4.start
  constraint coincident L2 L8.start
  constraint coincident L0 L8.end
  constraint perpendicular L0 L8
  constraint midpoint L0 L8.end
  constraint symmetric L5 L7 L8
  constraint horizontal L9
  constraint vertical L10
  constraint horizontal L11
  constraint vertical L12
  constraint equal L5 L6
  constraint equal L10 L11
  measures "d15" distance of L10.end L11.end
  measures "d17" horizontal distance of L6.end L11.end
  measures "d18" horizontal distance of L5.end L10.end
  measures "d29" distance of L6 L11
loft "Loft1" add profiles "Sketch2" section 1 face at (-5.7, 11, -14.6) section 2 contours L2 L4 L5 L6 L7 | L9 L10 L11 L12
extrude "Extrude3" cut sketch "Sketch2" against normal blind 30 contours L9 L10 L11 L12
sketch "Sketch3" plane through (0, 33, 0) normal (0, 1, 0) x (-1, 0, 0)
  line L0 (21.2, 10.1) -> (27.3, 10.1)
  line L1 (27.3, 10.1) -> (27.3, 7.9)
  line L2 (27.3, 7.9) -> (25.3, 7.9)
  line L3 (25.3, 7.9) -> (25.3, 5.7485)
  line L4 (25.3, 5.7485) -> (27.4485, 3.6)
  line L5 (27.4485, 3.6) -> (32.9515, 3.6)
  line L6 (32.9515, 3.6) -> (35.1, 5.7485)
  line L7 (35.1, 5.7485) -> (35.1, 7.9)
  line L8 (35.1, 7.9) -> (33.1, 7.9)
  line L9 (33.1, 7.9) -> (33.1, 10.1)
  line L10 (33.1, 10.1) -> (39.2, 10.1)
  arc A0 (40.3, 9) -> (39.2, 10.1) centre (39.2, 9) ccw
  line L11 (40.3, 9) -> (40.3, 2.9)
  line L12 (40.3, 2.9) -> (38.1, 2.9)
  line L13 (38.1, 2.9) -> (38.1, 4.9)
  line L14 (38.1, 4.9) -> (35.9485, 4.9)
  line L15 (35.9485, 4.9) -> (33.8, 2.7515)
  line L16 (33.8, 2.7515) -> (33.8, -2.7515)
  line L17 (33.8, -2.7515) -> (35.9485, -4.9)
  line L18 (35.9485, -4.9) -> (38.1, -4.9)
  line L19 (38.1, -4.9) -> (38.1, -2.9)
  line L20 (38.1, -2.9) -> (40.3, -2.9)
  line L21 (40.3, -2.9) -> (40.3, -9)
  arc A1 (39.2, -10.1) -> (40.3, -9) centre (39.2, -9) ccw
  line L22 (39.2, -10.1) -> (33.1, -10.1)
  line L23 (33.1, -10.1) -> (33.1, -7.9)
  line L24 (33.1, -7.9) -> (35.1, -7.9)
  line L25 (35.1, -7.9) -> (35.1, -5.7485)
  line L26 (35.1, -5.7485) -> (32.9515, -3.6)
  line L27 (32.9515, -3.6) -> (27.4485, -3.6)
  line L28 (27.4485, -3.6) -> (25.3, -5.7485)
  line L29 (25.3, -5.7485) -> (25.3, -7.9)
  line L30 (25.3, -7.9) -> (27.3, -7.9)
  line L31 (27.3, -7.9) -> (27.3, -10.1)
  line L32 (27.3, -10.1) -> (21.2, -10.1)
  arc A2 (20.1, -9) -> (21.2, -10.1) centre (21.2, -9) ccw
  line L33 (20.1, -9) -> (20.1, -2.9)
  line L34 (20.1, -2.9) -> (22.3, -2.9)
  line L35 (22.3, -2.9) -> (22.3, -4.9)
  line L36 (22.3, -4.9) -> (24.4515, -4.9)
  line L37 (24.4515, -4.9) -> (26.6, -2.7515)
  line L38 (26.6, -2.7515) -> (26.6, 2.7515)
  line L39 (26.6, 2.7515) -> (24.4515, 4.9)
  line L40 (24.4515, 4.9) -> (22.3, 4.9)
  line L41 (22.3, 4.9) -> (22.3, 2.9)
  line L42 (22.3, 2.9) -> (20.1, 2.9)
  line L43 (20.1, 2.9) -> (20.1, 9)
  arc A3 (21.2, 10.1) -> (20.1, 9) centre (21.2, 9) ccw
  line L44 (2.9, 10.1) -> (9, 10.1)
  arc A4 (10.1, 9) -> (9, 10.1) centre (9, 9) ccw
  line L45 (10.1, 9) -> (10.1, 2.9)
  line L46 (10.1, 2.9) -> (7.9, 2.9)
  line L47 (7.9, 2.9) -> (7.9, 4.9)
  line L48 (7.9, 4.9) -> (5.7485, 4.9)
  line L49 (5.7485, 4.9) -> (3.6, 2.7515)
  line L50 (3.6, 2.7515) -> (3.6, -2.7515)
  line L51 (3.6, -2.7515) -> (5.7485, -4.9)
  line L52 (5.7485, -4.9) -> (7.9, -4.9)
  line L53 (7.9, -4.9) -> (7.9, -2.9)
  line L54 (7.9, -2.9) -> (10.1, -2.9)
  line L55 (10.1, -2.9) -> (10.1, -9)
  arc A5 (9, -10.1) -> (10.1, -9) centre (9, -9) ccw
  line L56 (9, -10.1) -> (2.9, -10.1)
  line L57 (2.9, -10.1) -> (2.9, -7.9)
  line L58 (2.9, -7.9) -> (4.9, -7.9)
  line L59 (4.9, -7.9) -> (4.9, -5.7485)
  line L60 (4.9, -5.7485) -> (2.7515, -3.6)
  line L61 (2.7515, -3.6) -> (-2.7515, -3.6)
  line L62 (-2.7515, -3.6) -> (-4.9, -5.7485)
  line L63 (-4.9, -5.7485) -> (-4.9, -7.9)
  line L64 (-4.9, -7.9) -> (-2.9, -7.9)
  line L65 (-2.9, -7.9) -> (-2.9, -10.1)
  line L66 (-2.9, -10.1) -> (-9, -10.1)
  arc A6 (-10.1, -9) -> (-9, -10.1) centre (-9, -9) ccw
  line L67 (-10.1, -9) -> (-10.1, -2.9)
  line L68 (-10.1, -2.9) -> (-7.9, -2.9)
  line L69 (-7.9, -2.9) -> (-7.9, -4.9)
  line L70 (-7.9, -4.9) -> (-5.7485, -4.9)
  line L71 (-5.7485, -4.9) -> (-3.6, -2.7515)
  line L72 (-3.6, -2.7515) -> (-3.6, 2.7515)
  line L73 (-3.6, 2.7515) -> (-5.7485, 4.9)
  line L74 (-5.7485, 4.9) -> (-7.9, 4.9)
  line L75 (-7.9, 4.9) -> (-7.9, 2.9)
  line L76 (-7.9, 2.9) -> (-10.1, 2.9)
  line L77 (-10.1, 2.9) -> (-10.1, 9)
  arc A7 (-9, 10.1) -> (-10.1, 9) centre (-9, 9) ccw
  line L78 (-9, 10.1) -> (-2.9, 10.1)
  line L79 (-2.9, 10.1) -> (-2.9, 7.9)
  line L80 (-2.9, 7.9) -> (-4.9, 7.9)
  line L81 (-4.9, 7.9) -> (-4.9, 5.7485)
  line L82 (-4.9, 5.7485) -> (-2.7515, 3.6)
  line L83 (-2.7515, 3.6) -> (2.7515, 3.6)
  line L84 (2.7515, 3.6) -> (4.9, 5.7485)
  line L85 (4.9, 5.7485) -> (4.9, 7.9)
  line L86 (4.9, 7.9) -> (2.9, 7.9)
  line L87 (2.9, 7.9) -> (2.9, 10.1)
  line L88 (43.3, -14.6) -> (43.3, 14.6)
  line L89 (43.3, 14.6) -> (-13.1, 14.6)
  line L90 (-13.1, 14.6) -> (-13.1, -14.6)
  line L91 (-13.1, -14.6) -> (2.1, -44.6)
  line L92 (2.1, -44.6) -> (28.1, -44.6)
  line L93 (28.1, -44.6) -> (43.3, -14.6)
  line L94 (15.1, -44.6) -> (15.1, -17.6132) construction
  circle A8 centre (15.1, -37.1) radius 2
  circle A9 centre (15.1, -22.1) radius 2
  dimension "d23" = 4
  dimension "d24" = 7.5
  dimension "d25" = 15
  constraint midpoint L92 L94.start
  constraint perpendicular L92 L94
  constraint coincident L94 A8.centre
  constraint coincident L94 A9.centre
  constraint equal A8 A9
  measures "d23" diameter of A8
  measures "d24" distance of L94.start A8.centre
  measures "d25" distance of A8.centre A9.centre
extrude "Extrude4" cut sketch "Sketch3" against normal blind 4 contours A8 | A9
equation "d15 = 20 mm + 2 * gap"
equation "d17 = 3 mm - gap"
equation "d18 = 3 mm - gap"
equation "gap = 0.2 mm"
equation "d29 = 3 mm - gap"

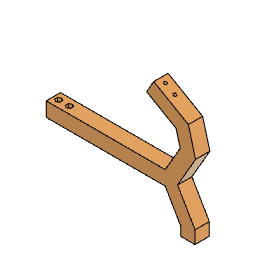
design "leg"
Autodesk Fusion 360 part; units mm, degrees
sketch "Sketch1" plane through (0, 0, 0) normal (0, 1, 0) x (1, 0, 0)
  line L0 (0, 0) -> (44.8288, 25.8819)
  line L1 (0, 0) -> (68.1027, 0) construction
  line L2 (44.8288, 25.8819) -> (52.6768, 55.1712)
  line L3 (52.6768, 55.1712) -> (26.7949, 100)
  line L4 (26.7949, 100) -> (52.6768, 144.8288)
  line L5 (26.7949, 100) -> (-145.5051, 100)
  line L6 (0, 0) -> (26.7949, 100) construction
  circle A0 centre (13.3975, 50) radius 36.6025 construction
  line L7 (52.6768, 144.8288) -> (52.6768, 160)
  dimension "d1" = 30
  dimension "d2" = 120
  dimension "d3" = 120
  dimension "d4" = 135
  dimension "d5" = 100
  dimension "d29" = 60
  dimension "d30" = 172.3
  constraint coincident L0.start L1.start
  constraint horizontal L1
  constraint horizontal L5
  constraint equal L0 L3
  constraint midpoint L6 A0.centre
  constraint tangent L0 A0
  constraint tangent L2 A0
  constraint vertical L2.end L4.end
  constraint vertical L7
  measures "d1" angle of L0 L1
  measures "d2" angle of L3 L4
  measures "d3" angle of L4 L5
  measures "d4" angle of L0 L2
  measures "d5" distance of L0.start L5
  measures "d29" distance of L5 L7.end
  measures "d30" distance of L3.end L5.end
pipe "Pipe1" add square section size 20 path "Sketch1" along L0 L2 L3 L4 L7
pipe "Pipe2" add square section size 20 path "Sketch1" along L5
sketch "Sketch2" plane through (5, 0, 8.6603) normal (0.5, 0, 0.866025) x (0, 1, 0)
  line L0 (10, 0) -> (-10, 0)
  line L1 (-10, 0) -> (-10, -55.9059)
  line L2 (-10, -55.9059) -> (10, -55.9059)
  line L3 (10, -55.9059) -> (10, 0)
  line L4 (0, 0) -> (0, -55.9059) construction
  circle A0 centre (0, -7.5) radius 2
  circle A1 centre (0, -22.5) radius 2
  line L5 (2.1362, -3.8) -> (-2.1362, -3.8)
  line L6 (-2.1362, -3.8) -> (-4.2724, -7.5)
  line L7 (-4.2724, -7.5) -> (-2.1362, -11.2)
  line L8 (-2.1362, -11.2) -> (2.1362, -11.2)
  line L9 (2.1362, -11.2) -> (4.2724, -7.5)
  line L10 (4.2724, -7.5) -> (2.1362, -3.8)
  line L11 (2.1362, -18.8) -> (-2.1362, -18.8)
  line L12 (-2.1362, -18.8) -> (-4.2724, -22.5)
  line L13 (-4.2724, -22.5) -> (-2.1362, -26.2)
  line L14 (-2.1362, -26.2) -> (2.1362, -26.2)
  line L15 (2.1362, -26.2) -> (4.2724, -22.5)
  line L16 (4.2724, -22.5) -> (2.1362, -18.8)
  point P0 (0, -7.5)
  point P1 (0, -22.5)
  dimension "d14" = 4
  dimension "d15" = 7.5
  dimension "d16" = 15
  dimension "d19" = 7.4
  constraint coincident L4.start origin
  constraint midpoint L2 L4.end
  constraint coincident L4 P0
  constraint coincident L4 P1
  constraint equal A0 A1
  constraint coincident P0 A0.centre
  constraint coincident P1 A1.centre
  constraint horizontal L5.start L5.end
  constraint horizontal L11
  constraint vertical L9.end L15.end
  measures "d14" diameter of A0
  measures "d15" distance of L4.start A0.centre
  measures "d16" distance of P0 P1
  measures "d19" distance of L5.start L8.end
extrude "Extrude1" cut sketch "Sketch2" against normal blind 35 contours A0 | A1
extrude "Extrude2" cut sketch "Sketch2" along normal blind 5 from surface at -20 contours L5 L6 L7 L8 L9 L10 | L11 L12 L13 L14 L15 L16